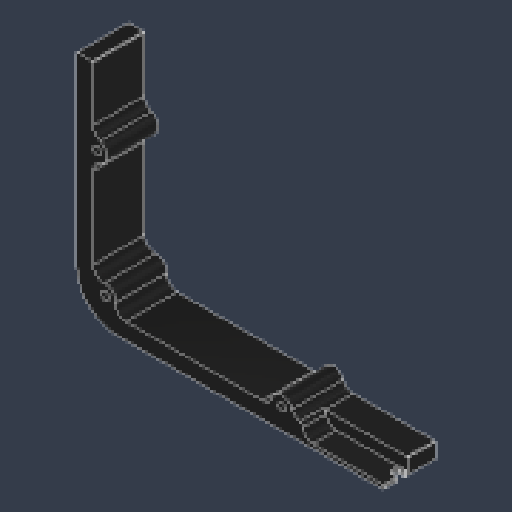
# Autodesk Inventor part: Corner Top Right
Saved by Autodesk Inventor 2023.4 (Build 274418000, 418)
## iProperties
Created: 2024-02-24
Part Number: Corner Top Right
Material: Generic
Document SubType Name: Modeling
Designer: JoaoSilva
Density: 1 g/cm^3
Appearance: Smooth - Black
Author: JoaoSilva
Autodesk Inventor part; units mm, degrees
ref_plane "YZ Plane" through (0, 0, 0) normal (1, 0, 0) x (0, 1, 0)
ref_plane "XZ Plane" through (0, 0, 0) normal (0, 1, 0) x (-1, 0, 0)
ref_plane "XY Plane" through (0, 0, 0) normal (0, 0, 1) x (1, 0, 0)
sketch "Sketch1" plane through (0, 0, 0) normal (0, 0, 1) x (1, 0, 0)
  line L0 (-74.8, 54.8) -> (74.8, 54.8)
  line L1 (74.8, 54.8) -> (74.8, -54.8)
  line L2 (74.8, -54.8) -> (-74.8, -54.8)
  line L3 (-74.8, -54.8) -> (-74.8, 54.8)
  line L4 (-74.8, 54.8) -> (74.8, -54.8) construction
  line L5 (74.8, 54.8) -> (-74.8, -54.8) construction
  line L6 (-66.8, 54.8) -> (-66.8, -46.8)
  line L7 (-66.8, -46.8) -> (74.8, -46.8)
  point P0 (0, 0)
  dimension "d0" = 149.6
  dimension "d1" = 109.6
  dimension "d2" = 8
  dimension "d3" = 8
  constraints: 16 end point, 3 perpendicular, 2 midpoint, 2 parallel, 2 point on line, 1 horizontal
  measures "d0" distance of L1.end L2.end
  measures "d1" distance of L2.end L0.start
  measures "d2" distance between parallel lines of L2 L7
  measures "d3" distance between parallel lines of L3 L6
extrude "Extrusion1" add sketch "Sketch1" along normal blind 25 contours L0 L6 L7 L1 L2 L3
fillet "Fillet1" radius 12 1 edges at (-66.8, -46.8, 12.5)
fillet "Fillet2" radius 20 1 edges at (-74.8, -54.8, 12.5)
sketch "Sketch2" plane through (0, 0, 25) normal (0, 0, 1) x (1, 0, 0)
  circle A0 centre (25.2, -44.8) radius 5
  circle A1 centre (-60.8, -40.8) radius 5
  circle A2 centre (-64.8, 18.2) radius 5
  line L0 (-54.8, -54.8) -> (74.8, -54.8) projected
  line L1 (-74.8, 54.8) -> (-74.8, -34.8) projected
  point P0 (0, 0)
  dimension "d8" = 10
  dimension "d9" = 10
  dimension "d10" = 14
  dimension "d11" = 14
  dimension "d12" = 73
  dimension "d13" = 100
  dimension "d14" = 10
  constraints: 3 centre point, 2 equal radius
  measures "d8" distance from line of L0 A0.centre
  measures "d9" distance from line of L1 A2.centre
  measures "d10" distance from line of L0 A1.centre
  measures "d11" distance from line of L1 A1.centre
  measures "d12" distance from line of L0 A2.centre
  measures "d13" distance from line of A0.centre L1
  measures "d14" diameter of A0
extrude "Extrusion2" add sketch "Sketch2" against normal up to surface (25 mm away)
sketch "Sketch3" plane through (0, 0, 25) normal (0, 0, 1) x (1, 0, 0)
  arc A0 (-66.8, 13.6174) -> (-66.8, 22.7826) centre (-64.8, 18.2) ccw projected
  arc A1 (-59.8147, -45.702) -> (-65.702, -39.8147) centre (-60.8, -40.8) ccw projected
  arc A2 (29.7826, -46.8) -> (20.6174, -46.8) centre (25.2, -44.8) ccw projected
  point P0 (0, 0)
hole "Hole1" at (-64.8, 18.2, 25) at (-60.8, -40.8, 25) at (25.2, -44.8, 25) direction (0, 0, -1) diameter 4 end through all
fillet "Fillet3" radius 5 6 edges at (29.7826, -46.8, 12.5) (20.6174, -46.8, 12.5) (-65.702, -39.8147, 12.5) (-59.8147, -45.702, 12.5) (-66.8, 22.7826, 12.5) (-66.8, 13.6174, 12.5)
fillet "Fillet4" radius 0.4 4 edges at (-74.8, 54.8, 12.5) (-66.8, 54.8, 12.5) (74.8, -54.8, 12.5) (74.8, -46.8, 12.5)
sketch "Sketch4" plane through (34.7394, -46.8, 25) normal (0, 1, 0) x (1, 0, 0)
  line L0 (40.0606, 0) -> (0.4606, 0)
  line L1 (0.4606, 0) -> (0.4606, 11.4)
  line L2 (0.4606, 11.4) -> (40.0606, 11.4)
  line L3 (40.0606, 11.4) -> (40.0606, 0)
  line L4 (-109.5394, 25) -> (-109.5394, 0) projected
  line L5 (39.6606, 25) -> (0, 25) projected
  line L6 (40.0606, 0) -> (40.0606, 25) projected
  line L7 (39.6606, 0) -> (0, 0) projected
  point P0 (-34.7394, 25)
  dimension "d26" = 110
  dimension "d27" = 13.6
  constraints: 8 end point, 2 collinear, 2 parallel, 1 horizontal, 1 perpendicular
  measures "d26" distance between parallel lines of L4 L1
  measures "d27" distance between parallel lines of L5 L2
extrude "Extrusion3" cut sketch "Sketch4" against normal blind 6
sketch "Sketch5" plane through (34.7394, -46.8, 25) normal (0, 1, 0) x (1, 0, 0)
  line L0 (43.4606, 8.4) -> (37.4606, 8.4) construction
  line L1 (43.4606, 10) -> (37.4606, 10)
  line L2 (37.4606, 6.8) -> (43.4606, 6.8)
  arc A0 (43.4606, 6.8) -> (43.4606, 10) centre (43.4606, 8.4) ccw
  arc A1 (37.4606, 10) -> (37.4606, 6.8) centre (37.4606, 8.4) ccw
  line L3 (40.0606, 11.4) -> (40.0606, 0) projected
  line L4 (39.6606, 25) -> (0, 25) projected
  point P0 (-34.7394, 25)
  point P1 (40.4606, 8.4)
  point P2 (45.0606, 8.4)
  point P3 (35.8606, 8.4)
  dimension "d31" = 0.4
  dimension "d32" = 3.2
  dimension "d33" = 16.6
  dimension "d35" = 9.2
  constraints: 8 end point, 6 point on circle, 4 tangent, 2 centre point, 1 horizontal, 1 midpoint, 1 parallel
  measures "d31" distance from line of L3 point (40.461, 8.4)
  measures "d32" distance between parallel lines of L1 L2
  measures "d33" distance between parallel lines of L4 L0
  measures "d35" distance of point (45.061, 8.4) point (35.861, 8.4)
extrude "Extrusion4" cut sketch "Sketch5" against normal through all
fillet "Fillet5" radius 0.4 2 edges at (74.8, -52.8, 14.3) (74.8, -52.8, 21.6)
fillet "Fillet6" radius 0.4 12 edges at (74.6828, -52.9172, 18.2) (73.3, -52.8, 18.2) (70.6, -52.8, 16.6) (73.3, -52.8, 15) (74.6828, -52.9172, 15) (74.8, -53.8, 15) (74.6828, -54.6828, 15) (73.3, -54.8, 15) (70.6, -54.8, 16.6) (73.3, -54.8, 18.2) (74.6828, -54.6828, 18.2) (74.8, -53.8, 18.2)
fillet "Fillet7" radius 2 1 edges at (35.2, -46.8, 19.3)
fillet "Fillet8" radius 5 1 edges at (35.2, -52.8, 19.3)
equation "\"d3\" = d2"
equation "\"d9\" = d8"
equation "\"d11\" = d10"
body "Solid1"
